Autodesk Inventor part; units mm, degrees
(part 2 of 2)
  line L135 (29.2243, -208.6026) -> (30.7211, -208.6026)
  line L136 (30.7211, -208.6026) -> (30.7211, -208.9558)
  spline S178 degree 2 poles (33.0256, -207.4318) (33.0256, -208.2519) (32.5489, -209.02) (32.0524, -209.02) knots 0 0 0 1 2 2 2
  spline S179 degree 2 poles (32.0524, -209.02) (31.5486, -209.02) (31.0768, -208.237) (31.0768, -207.4343) knots 0 0 0 1 2 2 2
  spline S180 degree 2 poles (31.0768, -207.4343) (31.0768, -206.6093) (31.5535, -205.8461) (32.0524, -205.8461) knots 0 0 0 1 2 2 2
  spline S181 degree 2 poles (32.0524, -205.8461) (32.5539, -205.8461) (33.0256, -206.6365) (33.0256, -207.4318) knots 0 0 0 1 2 2 2
  spline S182 degree 2 poles (32.502, -208.3605) (32.5613, -208.2099) (32.6107, -207.7455) (32.6107, -207.4318) knots 0 0 0 1 2 2 2
  spline S183 degree 2 poles (32.6107, -207.4318) (32.6107, -207.1181) (32.5613, -206.6562) (32.4995, -206.5006) knots 0 0 0 1 2 2 2
  spline S184 degree 2 poles (32.4995, -206.5006) (32.4378, -206.345) (32.2229, -206.1845) (32.0524, -206.1845) knots 0 0 0 1 2 2 2
  spline S185 degree 2 poles (32.0524, -206.1845) (31.882, -206.1845) (31.6622, -206.345) (31.598, -206.5056) knots 0 0 0 1 2 2 2
  spline S186 degree 2 poles (31.598, -206.5056) (31.5362, -206.6612) (31.4917, -207.1354) (31.4917, -207.4343) knots 0 0 0 1 2 2 2
  spline S187 degree 2 poles (31.4917, -207.4343) (31.4917, -207.7554) (31.5313, -208.1852) (31.5955, -208.3531) knots 0 0 0 1 2 2 2
  spline S188 degree 2 poles (31.5955, -208.3531) (31.6548, -208.5112) (31.8746, -208.6816) (32.0524, -208.6816) knots 0 0 0 1 2 2 2
  spline S189 degree 2 poles (32.0524, -208.6816) (32.2204, -208.6816) (32.4402, -208.5211) (32.502, -208.3605) knots 0 0 0 1 2 2 2
  line L137 (35.2956, -208.9558) -> (33.4159, -208.9558)
  line L138 (33.4159, -208.9558) -> (33.4159, -208.5236)
  spline S190 degree 2 poles (33.4159, -208.5236) (33.6184, -208.3334) (33.9791, -207.9802) (34.152, -207.79) knots 0 0 0 1 2 2 2
  spline S191 degree 2 poles (34.152, -207.79) (34.5002, -207.4071) (34.7546, -206.9477) (34.7546, -206.7032) knots 0 0 0 1 2 2 2
  spline S192 degree 2 poles (34.7546, -206.7032) (34.7546, -206.5747) (34.6756, -206.3821) (34.604, -206.3203) knots 0 0 0 1 2 2 2
  spline S193 degree 2 poles (34.604, -206.3203) (34.5323, -206.2586) (34.3446, -206.1968) (34.231, -206.1968) knots 0 0 0 1 2 2 2
  spline S194 degree 2 poles (34.231, -206.1968) (34.1223, -206.1968) (33.9, -206.2512) (33.7987, -206.2931) knots 0 0 0 1 2 2 2
  spline S195 degree 2 poles (33.7987, -206.2931) (33.7123, -206.3277) (33.5517, -206.4265) (33.5023, -206.4611) knots 0 0 0 1 2 2 2
  line L139 (33.5023, -206.4611) -> (33.4801, -206.4611)
  line L140 (33.4801, -206.4611) -> (33.4801, -206.0264)
  spline S196 degree 2 poles (33.4801, -206.0264) (33.6061, -205.9646) (34.0581, -205.8436) (34.2606, -205.8436) knots 0 0 0 1 2 2 2
  spline S197 degree 2 poles (34.2606, -205.8436) (34.6879, -205.8436) (35.1696, -206.2956) (35.1696, -206.6809) knots 0 0 0 1 2 2 2
  spline S198 degree 2 poles (35.1696, -206.6809) (35.1696, -206.8612) (35.0856, -207.1626) (35.0115, -207.291) knots 0 0 0 1 2 2 2
  spline S199 degree 2 poles (35.0115, -207.291) (34.9374, -207.4244) (34.7225, -207.6862) (34.604, -207.8122) knots 0 0 0 1 2 2 2
  spline S200 degree 2 poles (34.604, -207.8122) (34.4113, -208.0222) (33.9395, -208.4717) (33.7987, -208.6026) knots 0 0 0 1 2 2 2
  line L141 (33.7987, -208.6026) -> (35.2956, -208.6026)
  line L142 (35.2956, -208.6026) -> (35.2956, -208.9558)
  spline S201 degree 2 poles (37.6297, -207.9678) (37.6297, -208.2025) (37.4741, -208.6001) (37.3432, -208.7335) knots 0 0 0 1 2 2 2
  spline S202 degree 2 poles (37.3432, -208.7335) (37.2074, -208.8743) (36.8665, -209.02) (36.6615, -209.02) knots 0 0 0 1 2 2 2
  spline S203 degree 2 poles (36.6615, -209.02) (36.4565, -209.02) (36.1181, -208.8817) (35.9896, -208.7434) knots 0 0 0 1 2 2 2
  spline S204 degree 2 poles (35.9896, -208.7434) (35.8316, -208.5779) (35.6537, -208.0222) (35.6537, -207.6171) knots 0 0 0 1 2 2 2
  spline S205 degree 2 poles (35.6537, -207.6171) (35.6537, -207.2194) (35.8167, -206.5797) (35.9872, -206.3425) knots 0 0 0 1 2 2 2
  spline S206 degree 2 poles (35.9872, -206.3425) (36.1527, -206.1104) (36.6763, -205.851) (37.0196, -205.851) knots 0 0 0 1 2 2 2
  spline S207 degree 2 poles (37.0196, -205.851) (37.1209, -205.851) (37.2988, -205.8708) (37.3654, -205.893) knots 0 0 0 1 2 2 2
  line L143 (37.3654, -205.893) -> (37.3654, -206.2857)
  line L144 (37.3654, -206.2857) -> (37.3482, -206.2857)
  spline S208 degree 2 poles (37.3482, -206.2857) (37.2913, -206.2561) (37.0839, -206.2042) (36.9653, -206.2042) knots 0 0 0 1 2 2 2
  spline S209 degree 2 poles (36.9653, -206.2042) (36.5849, -206.2042) (36.1181, -206.718) (36.0736, -207.2219) knots 0 0 0 1 2 2 2
  spline S210 degree 2 poles (36.0736, -207.2219) (36.2194, -207.1206) (36.5256, -207.0094) (36.7084, -207.0094) knots 0 0 0 1 2 2 2
  spline S211 degree 2 poles (36.7084, -207.0094) (36.8863, -207.0094) (37.153, -207.0811) (37.2988, -207.1898) knots 0 0 0 1 2 2 2
  spline S212 degree 2 poles (37.2988, -207.1898) (37.4667, -207.3157) (37.6297, -207.706) (37.6297, -207.9678) knots 0 0 0 1 2 2 2
  spline S213 degree 2 poles (37.2148, -207.9851) (37.2148, -207.7974) (37.116, -207.543) (37.0073, -207.454) knots 0 0 0 1 2 2 2
  spline S214 degree 2 poles (37.0073, -207.454) (36.9258, -207.3898) (36.7232, -207.3478) (36.617, -207.3478) knots 0 0 0 1 2 2 2
  spline S215 degree 2 poles (36.617, -207.3478) (36.4738, -207.3478) (36.2045, -207.4343) (36.0736, -207.5158) knots 0 0 0 1 2 2 2
  spline S216 degree 2 poles (36.0736, -207.5158) (36.0712, -207.5603) (36.0662, -207.6442) (36.0662, -207.7085) knots 0 0 0 1 2 2 2
  spline S217 degree 2 poles (36.0662, -207.7085) (36.0662, -208.0246) (36.1897, -208.4124) (36.2836, -208.5137) knots 0 0 0 1 2 2 2
  spline S218 degree 2 poles (36.2836, -208.5137) (36.37, -208.61) (36.5578, -208.6866) (36.664, -208.6866) knots 0 0 0 1 2 2 2
  spline S219 degree 2 poles (36.664, -208.6866) (36.911, -208.6866) (37.2148, -208.3358) (37.2148, -207.9851) knots 0 0 0 1 2 2 2
  point P0 (0, 0)
  constraints: 2 other
emboss "Emboss1" sketch "Sketch14" operation cut depth 2.54 direction (-1, 0, 0)
sketch "Sketch16" plane through (5.08, 0, 0) normal (1, 0, 0) x (0, 0, -1)
  line L0 (-41.7074, -74.9522) -> (39.5726, -74.9522)
  line L1 (39.5726, -74.9522) -> (39.5726, -78.7622)
  line L2 (39.5726, -78.7622) -> (-41.7074, -78.7622)
  line L3 (-41.7074, -78.7622) -> (-41.7074, -74.9522)
  line L4 (22.7938, -210.0802) -> (-43.6417, -210.0802) projected
  point P0 (0, 0)
  point P1 (-43.6417, -212.6202)
  dimension "d193" = 135.128
  dimension "d195" = 3.81
  constraints: 8 end point, 2 parallel, 1 horizontal, 1 perpendicular
  measures "d193" distance between parallel lines of L4 L0
  measures "d195" distance between parallel lines of L0 L2
extrude "Extrusion13" add sketch "Sketch16" along normal blind 5.08
sketch "Sketch17" plane through (20.32, 33.2264, 20.9087) normal (0, 1, 0) x (1, 0, 0)
  line L0 (-4.318, 35.56) -> (0, 35.56) projected
  line L1 (-0.0061, 35.56) -> (0.0392, 35.56)
  line L2 (0, 64.9986) -> (0, -27.9146) projected
  line L3 (0, 35.5801) -> (0, 35.5243)
  line L4 (5, -24.7396) -> (5, 61.8236) projected
  line L5 (0, 35.56) -> (5, 35.56)
  line L6 (5, 35.56) -> (5, -0.0031)
  line L7 (5, -0.0031) -> (0, -0.0031)
  line L8 (0, -0.0031) -> (0, 35.56)
  point P0 (-20.32, 20.9087)
  point P1 (5, -23.8506)
  point P2 (5, 69.0626)
  point P3 (0.0392, 35.56)
  constraints: 12 end point, 4 point on line, 2 horizontal, 2 parallel, 1 perpendicular
extrude "Extrusion14" cut sketch "Sketch17" against normal blind 2.0066
sketch "Sketch18" plane through (0, 0, 0) normal (-1, 0, 0) x (0, 0, 1)
  arc A0 (46.2144, 33.1755) -> (48.7724, 30.6175) centre (48.0867, 32.4898) ccw projected
  circle A1 centre (48.0867, 32.4898) radius 4.5085
  arc A2 (-41.481, 33.1755) -> (-44.039, 30.6175) centre (-43.3533, 32.4898) ccw projected
  circle A3 centre (-43.3533, 32.4898) radius 4.5085
  arc A4 (-44.039, -212.018) -> (-41.481, -214.576) centre (-43.3533, -213.8902) ccw projected
  circle A5 centre (-43.3533, -213.8902) radius 4.5085
  arc A6 (46.2144, -214.576) -> (48.7724, -212.018) centre (48.0867, -213.8902) ccw projected
  circle A7 centre (48.0867, -213.8902) radius 4.5085
  point P0 (0, 0)
  dimension "d209" = 9.017
  dimension "d210" = 9.017
  dimension "d211" = 9.017
  dimension "d212" = 9.017
  constraints: 4 centre point, 4 coincident
  measures "d209" diameter of A1
  measures "d210" diameter of A3
  measures "d211" diameter of A5
  measures "d212" diameter of A7
extrude "Extrusion15" [suppressed]
sketch "Sketch19" plane through (20.32, -68.6784, -44.0899) normal (0, 0, -1) x (-1, 0, 0)
  line L0 (3.81, 0) -> (0, 0) projected
  line L1 (-5, 96.7232) -> (-5, -140.7668) projected
  line L2 (0, 0) -> (-5, 0)
  line L3 (-5, 0) -> (-5, 8.001)
  line L4 (-5, 8.001) -> (0, 8.001)
  line L5 (0, 8.001) -> (0, 0)
  point P0 (20.32, 68.6784)
  dimension "d216" = 5
  dimension "d219" = 8.001
  constraints: 8 end point, 2 parallel, 1 horizontal, 1 perpendicular, 1 point on line
  measures "d216" distance between parallel lines of L1 L5
  measures "d219" distance between parallel lines of L2 L4
extrude "Extrusion16" cut sketch "Sketch19" against normal blind 24.13
sketch "Sketch20" plane through (0, 0, 0) normal (-1, 0, 0) x (0, 0, 1)
  line L0 (41.2351, -52.8796) -> (44.7657, -52.8796)
  line L1 (44.7657, -52.8796) -> (46.8041, -56.4102)
  line L2 (41.2351, -52.8796) -> (39.1967, -56.4102)
  line L3 (44.7657, -59.9408) -> (46.8041, -56.4102)
  line L4 (41.2351, -59.9408) -> (39.1967, -56.4102)
  line L5 (41.2351, -59.9408) -> (44.7657, -59.9408)
  line L6 (-40.0449, -52.8796) -> (-36.5143, -52.8796)
  line L7 (-36.5143, -52.8796) -> (-34.4759, -56.4102)
  line L8 (-40.0449, -52.8796) -> (-42.0833, -56.4102)
  line L9 (-36.5143, -59.9408) -> (-34.4759, -56.4102)
  line L10 (-40.0449, -59.9408) -> (-42.0833, -56.4102)
  line L11 (-40.0449, -59.9408) -> (-36.5143, -59.9408)
  line L12 (-45.1249, 28.9592) -> (-41.5943, 28.9592)
  line L13 (-45.1249, 36.0204) -> (-41.5943, 36.0204)
  line L14 (-45.1249, 28.9592) -> (-47.1633, 32.4898)
  line L15 (-45.1249, 36.0204) -> (-47.1633, 32.4898)
  line L16 (-41.5943, 28.9592) -> (-39.5559, 32.4898)
  line L17 (-41.5943, 36.0204) -> (-39.5559, 32.4898)
  line L18 (49.8457, 36.0204) -> (51.8841, 32.4898)
  line L19 (49.8457, 28.9592) -> (51.8841, 32.4898)
  line L20 (46.3151, 28.9592) -> (49.8457, 28.9592)
  line L21 (46.3151, 36.0204) -> (49.8457, 36.0204)
  line L22 (46.3151, 36.0204) -> (44.2767, 32.4898)
  line L23 (46.3151, 28.9592) -> (44.2767, 32.4898)
  line L24 (-41.5943, -210.3596) -> (-39.5559, -213.8902)
  line L25 (-41.5943, -217.4208) -> (-39.5559, -213.8902)
  line L26 (-45.1249, -217.4208) -> (-41.5943, -217.4208)
  line L27 (-45.1249, -210.3596) -> (-41.5943, -210.3596)
  line L28 (-45.1249, -210.3596) -> (-47.1633, -213.8902)
  line L29 (-45.1249, -217.4208) -> (-47.1633, -213.8902)
  line L30 (49.8457, -210.3596) -> (51.8841, -213.8902)
  line L31 (49.8457, -217.4208) -> (51.8841, -213.8902)
  line L32 (46.3151, -217.4208) -> (49.8457, -217.4208)
  line L33 (46.3151, -210.3596) -> (49.8457, -210.3596)
  line L34 (46.3151, -210.3596) -> (44.2767, -213.8902)
  line L35 (46.3151, -217.4208) -> (44.2767, -213.8902)
  point P0 (0, 0)
  point P1 (43.0004, -59.9408)
  point P2 (-38.2796, -59.9408)
  point P3 (-38.2733, -56.4102)
  point P4 (-43.3596, 28.9592)
  point P5 (-43.3533, 32.4898)
  point P6 (48.0804, 28.9592)
  point P7 (-43.3596, -217.4208)
  point P8 (48.0804, -217.4208)
  dimension "d332" = 7.0612
  dimension "d333" = 120
  dimension "d334" = 120
  dimension "d335" = 120
  dimension "d336" = 120
  dimension "d337" = 3.5306
  dimension "d338" = 3.5306
  dimension "d339" = 3.5306
  dimension "d340" = 3.5306
  dimension "d341" = 3.5306
  dimension "d342" = 3.5306
  dimension "d343" = 0
  dimension "d344" = 7.6074
  dimension "d349" = 7.0612
  dimension "d350" = 120
  dimension "d351" = 120
  dimension "d352" = 120
  dimension "d353" = 120
  dimension "d354" = 3.5306
  dimension "d355" = 3.5306
  dimension "d356" = 3.5306
  dimension "d357" = 3.5306
  dimension "d358" = 3.5306
  dimension "d359" = 3.5306
  dimension "d360" = 0
  dimension "d361" = 7.6074
  dimension "d366" = 7.0612
  dimension "d367" = 120
  dimension "d368" = 120
  dimension "d369" = 120
  dimension "d370" = 120
  dimension "d371" = 3.5306
  dimension "d372" = 3.5306
  dimension "d373" = 3.5306
  dimension "d374" = 3.5306
  dimension "d375" = 3.5306
  dimension "d376" = 3.5306
  dimension "d377" = 0
  dimension "d378" = 7.6074
  dimension "d383" = 7.0612
  dimension "d384" = 120
  dimension "d385" = 120
  dimension "d386" = 120
  dimension "d387" = 120
  dimension "d388" = 3.5306
  dimension "d389" = 3.5306
  dimension "d390" = 3.5306
  dimension "d391" = 3.5306
  dimension "d392" = 3.5306
  dimension "d393" = 3.5306
  dimension "d394" = 0
  dimension "d395" = 7.6074
  dimension "d402" = 7.0612
  dimension "d403" = 120
  dimension "d404" = 120
  dimension "d405" = 120
  dimension "d406" = 120
  dimension "d407" = 3.5306
  dimension "d408" = 3.5306
  dimension "d409" = 3.5306
  dimension "d410" = 3.5306
  dimension "d411" = 3.5306
  dimension "d412" = 3.5306
  dimension "d413" = 0
  constraints: 72 end point, 12 horizontal, 6 midpoint
  measures "d332" distance from line of point (43, -59.941) L0
  measures "d333" angle of L5 L4
  measures "d334" angle of L0 L2
  measures "d335" angle of L3 L5
  measures "d336" angle of L1 L0
  measures "d337" distance of L4.start L5.end
  measures "d338" distance of L2.start L0.end
  measures "d339" vertical distance of L2.start L2.end
  measures "d340" vertical distance of L4.start L4.end
  measures "d341" vertical distance of L0.end L1.end
  measures "d342" vertical distance of L5.end L3.end
  measures "d343" horizontal distance of L4.start L2.start
  measures "d344" distance of L3.end L4.end
  measures "d349" distance from line of point (-38.28, -59.941) L6
  measures "d350" angle of L11 L10
  measures "d351" angle of L6 L8
  measures "d352" angle of L9 L11
  measures "d353" angle of L7 L6
  measures "d354" distance of L10.start L11.end
  measures "d355" distance of L8.start L6.end
  measures "d356" vertical distance of L8.start L8.end
  measures "d357" vertical distance of L10.start L10.end
  measures "d358" vertical distance of L6.end L7.end
  measures "d359" vertical distance of L11.end L9.end
  measures "d360" horizontal distance of L10.start L8.start
  measures "d361" distance of L9.end L10.end
  measures "d366" distance from line of point (-43.36, 28.959) L13
  measures "d367" angle of L12 L14
  measures "d368" angle of L13 L15
  measures "d369" angle of L16 L12
  measures "d370" angle of L17 L13
  measures "d371" distance of L12.start L16.start
  measures "d372" distance of L13.start L17.start
  measures "d373" vertical distance of L13.start L15.end
  measures "d374" vertical distance of L12.start L14.end
  measures "d375" vertical distance of L17.start L17.end
  measures "d376" vertical distance of L16.start L16.end
  measures "d377" horizontal distance of L12.start L13.start
  measures "d378" distance of L16.end L14.end
  measures "d383" distance from line of point (48.08, 28.959) L21
  measures "d384" angle of L20 L23
  measures "d385" angle of L21 L22
  measures "d386" angle of L19 L20
  measures "d387" angle of L18 L21
  measures "d388" distance of L20.start L19.start
  measures "d389" distance of L21.start L18.start
  measures "d390" vertical distance of L21.start L22.end
  measures "d391" vertical distance of L20.start L23.end
  measures "d392" vertical distance of L18.start L18.end
  measures "d393" vertical distance of L19.start L19.end
  measures "d394" horizontal distance of L20.start L21.start
  measures "d395" distance of L19.end L23.end
  measures "d402" distance from line of point (-43.36, -217.421) L27
  measures "d403" angle of L26 L29
  measures "d404" angle of L27 L28
  measures "d405" angle of L25 L26
  measures "d406" angle of L24 L27
  measures "d407" distance of L26.start L25.start
  measures "d408" distance of L27.start L24.start
  measures "d409" vertical distance of L27.start L28.end
  measures "d410" vertical distance of L26.start L29.end
  measures "d411" vertical distance of L24.start L24.end
  measures "d412" vertical distance of L25.start L25.end
  measures "d413" horizontal distance of L26.start L27.start
extrude "Extrusion18" cut sketch "Sketch20" against normal blind 4
body "Solid1"
